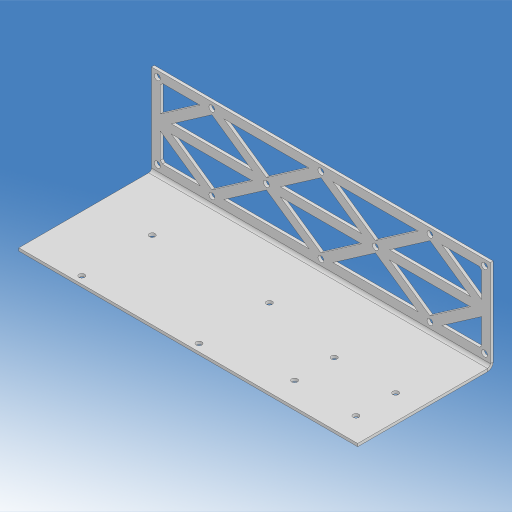
# Autodesk Inventor part: NEMA34_gearbox_sheetMetaMount
Saved by Autodesk Inventor 2024 (Build 280153000, 153)
## iProperties
Created: 2024-03-10
Part Number: NEMA34_gearbox_sheetMetaMount
Material: Generic
Document SubType Name: Sheet Metal
Designer: seene
Density: 1 g/cm^3
Sheet Metal Rule: Default
Appearance: Default
Author: seene
Autodesk Inventor part; units mm, degrees
(part 1 of 2)
ref_plane "YZ Plane" through (0, 0, 0) normal (1, 0, 0) x (0, 1, 0)
ref_plane "XZ Plane" through (0, 0, 0) normal (0, 1, 0) x (-1, 0, 0)
sketch "Sketch1" plane through (0, 0, 0) normal (0, 1, 0) x (-1, 0, 0)
  line L0 (0, 0) -> (144.145, 0) construction
  line L1 (144.145, 0) -> (144.145, -660.4) construction
  line L2 (144.145, -660.4) -> (0, -660.4) construction
  line L3 (0, -660.4) -> (0, 0) construction
  line L4 (144.145, -76.2) -> (0, -76.2) construction
  line L5 (144.145, -584.2) -> (0, -584.2) construction
  circle A0 centre (119.126, -452.5645) radius 3.175
  circle A1 centre (119.126, -519.1125) radius 3.175
  circle A2 centre (76.2, -519.1125) radius 3.175
  line L6 (55.753, -528.8044) -> (55.753, -436.6387) construction
  line L7 (139.573, -436.6387) -> (139.573, -528.8044) construction
  line L8 (55.753, -436.6387) -> (139.573, -436.6387) construction
  circle A3 centre (76.2, -452.5645) radius 3.175
  line L9 (139.573, -528.8044) -> (55.753, -528.8044) construction
  line L10 (92.9069, -436.6387) -> (102.4192, -436.6387) construction
  line L11 (102.4192, -412.6865) -> (92.9069, -412.6865) construction
  line L12 (92.9069, -412.6865) -> (92.9069, -436.6387) construction
  line L13 (97.663, -412.6865) -> (97.663, -436.6387) construction
  line L14 (102.4192, -436.6387) -> (102.4192, -412.6865) construction
  line L15 (89.7255, -412.623) -> (105.6005, -412.623) construction
  line L16 (140.97, -384.048) -> (54.356, -384.048) construction
  line L17 (105.6005, -384.048) -> (89.7255, -384.048) construction
  line L18 (89.7255, -384.048) -> (89.7255, -412.623) construction
  line L19 (97.663, -384.048) -> (97.663, -412.623) construction
  line L20 (105.6005, -412.623) -> (105.6005, -384.048) construction
  line L21 (140.97, -229.616) -> (140.97, -384.048) construction
  line L22 (54.356, -384.048) -> (54.356, -229.616) construction
  circle A4 centre (136.2075, -366.141) radius 3.175
  circle A5 centre (136.2075, -239.141) radius 3.175
  circle A6 centre (60.0075, -239.141) radius 3.175
  line L23 (54.356, -229.616) -> (140.97, -229.616) construction
  circle A7 centre (60.0075, -366.141) radius 3.175
  line L24 (144.145, -178.816) -> (0, -178.816)
  line L25 (0, -178.816) -> (0, -545.9494)
  line L26 (0, -545.9494) -> (144.145, -545.9494)
  line L27 (144.145, -545.9494) -> (144.145, -178.816)
  line L28 (139.573, -479.4885) -> (168.0972, -479.4885) construction
  line L29 (168.0972, -479.4885) -> (168.0972, -492.1885) construction
  line L30 (168.0972, -492.1885) -> (139.573, -492.1885) construction
  line L31 (139.573, -492.1885) -> (139.573, -479.4885) construction
  line L32 (168.0972, -485.8385) -> (139.573, -485.8385) construction
  line L33 (161.3624, -485.8385) -> (168.576, -485.8385) construction
  line L34 (136.4065, -431.8) -> (172.5514, -431.8) construction
  point P0 (89.7255, -398.3355)
  point P1 (72.0725, 0)
  point P2 (72.0725, -660.4)
  point P3 (72.0725, -178.816)
  point P4 (154.479, -431.8)
  dimension "d4" = 76.2
  dimension "d5" = 76.2
  dimension "d6" = 6.35
  dimension "d7" = 66.548
  dimension "d8" = 42.926
  dimension "d9" = 83.82
  dimension "d10" = 92.1657
  dimension "d11" = 20.447
  dimension "d12" = 15.9258
  dimension "d14" = 9.5123
  dimension "d16" = 23.9522
  dimension "d18" = 41.91
  dimension "d19" = 154.432
  dimension "d20" = 86.614
  dimension "d21" = 28.575
  dimension "d23" = 127
  dimension "d24" = 76.2
  dimension "d25" = 4.7625
  dimension "d26" = 9.525
  dimension "d27" = 15.875
  dimension "d28" = 144.145
  dimension "d29" = 660.4
  dimension "d30" = 6.35
  dimension "d116" = 28.5242
  dimension "d117" = 12.7
  dimension "d118" = 49.1998
  dimension "d122" = 50.8
  dimension "d123" = 17.145
  dimension "d126" = 0.0635
  dimension "d130" = 152.4
  dimension "d131" = 54.0385
  dimension "d490" = 3.175
  measures "d4" distance between parallel lines of L0 L4
  measures "d5" distance between parallel lines of L2 L5
  measures "d6" diameter of A0
  measures "d7" distance of A0.centre A1.centre
  measures "d8" distance of A0.centre A3.centre
  measures "d9" distance of L9.start L6.start
  measures "d10" distance of L6.start L8.start
  measures "d11" distance from line of L7 A0.centre
  measures "d12" distance from line of A0.centre L8
  measures "d14" distance of L11.start L11.end
  measures "d16" distance of L10.end L11.start
  measures "d18" distance between parallel lines of L7 L13
  measures "d19" distance of L23.end L21.end
  measures "d20" distance of L23.start L23.end
  measures "d21" distance of L15.end L17.start
  measures "d23" distance of A5.centre A4.centre
  measures "d24" distance of A5.centre A6.centre
  measures "d25" distance from line of L21 A5.centre
  measures "d26" distance from line of A6.centre L23
  measures "d27" distance from line of point (89.726, -398.336) L20
  measures "d28" distance between parallel lines of L3 L1
  measures "d29" distance from line of point (72.073, -660.4) L0
  measures "d30" diameter of A5
  measures "d116" distance of L29.end L30.end
  measures "d117" distance between parallel lines of L30 L28
  measures "d118" distance between parallel lines of L32 L8
  measures "d122" distance between parallel lines of L23 L24
  measures "d123" distance between parallel lines of L26 L9
  measures "d126" distance between parallel lines of L11 L15
  measures "d130" distance between parallel lines of L5 L34
  measures "d131" distance between parallel lines of L32 L34
  measures "d490" distance between parallel lines of L27 L21
extrude "Plate1" add sketch "Sketch1" along normal blind 3.048
ref_plane "Work Plane1" through (6.35, 0, -178.816) normal (1, 0, 0) x (0, 0, -1)
sketch "Sketch2" plane through (6.35, 0, -178.816) normal (1, 0, 0) x (0, 0, -1)
  line L0 (367.1334, 3.048) -> (0, 3.048) projected
  line L1 (0, 0) -> (0, 3.048) projected
  line L2 (0, 0) -> (367.1334, 0) projected
  line L3 (367.1334, 0) -> (367.1334, 3.048) projected
  line L4 (367.1334, 0) -> (0, 0)
  line L5 (0, 0) -> (0, -85.852)
  line L6 (0, -85.852) -> (367.1334, -85.852)
  line L7 (367.1334, -85.852) -> (367.1334, 0)
  point P0 (-178.816, 0)
  dimension "d132" = 88.9
  constraints: 8 end point, 2 parallel, 1 horizontal, 1 perpendicular
  measures "d132" distance between parallel lines of L0 L6
sketch "Sketch3" plane through (0, 0, 0) normal (0, -1, 0) x (1, 0, 0)
  line L0 (0, -178.816) -> (0, -545.9494) projected
  line L1 (0, -545.9494) -> (88.9, -545.9494)
  line L2 (88.9, -545.9494) -> (88.9, -178.816)
  line L3 (88.9, -178.816) -> (0, -178.816)
  line L4 (0, -178.816) -> (0, -545.9494)
  line L5 (0, -545.9494) -> (0, -178.816)
  point P0 (0, 0)
  point P1 (0, -138.2272)
  dimension "d50" = 88.9
  constraints: 10 end point, 3 equal length, 1 horizontal, 1 perpendicular
  measures "d50" distance of L0.start L2.end
sheet face with bend "Face2" sketch "Sketch3" thickness 3.048 toward (0, 1, 0) bend radius 3.048
bend "Bend1"
fold "Fold1" angle 90 bend radius 3.048 thickness 3.048 k factor 0.44 line from (0, 0, -178.816) to (0, 0, -545.9494) line at bend centre moving side (1, 0, 0) folds toward (0, -1, 0)
sketch "Sketch4" plane through (-0.3992, -88.5008, -545.9494) normal (-1, 0, 0) x (0, 0, 1)
  line L0 (367.1334, 85.4528) -> (0, 85.4528) projected
  line L1 (0, 85.4528) -> (0, 0) projected
  line L2 (0, 0) -> (367.1334, 0) projected
  line L3 (367.1334, 0) -> (409.19, 0)
  line L4 (409.19, 0) -> (409.19, 148.9528)
  line L5 (409.19, 148.9528) -> (367.1334, 148.9528)
  line L6 (367.1334, 148.9528) -> (367.1334, 0)
  line L7 (0, 0) -> (-42.7389, 0)
  line L8 (-42.7389, 0) -> (-42.7389, 148.9528)
  line L9 (-42.7389, 148.9528) -> (0, 148.9528)
  line L10 (0, 148.9528) -> (0, 0)
  line L11 (367.1334, 0) -> (-39.2666, 0)
  line L12 (367.1334, 85.4528) -> (367.1334, 0) projected
  point P0 (545.9494, 88.5008)
  constraints: 18 end point, 4 parallel, 3 horizontal, 2 perpendicular
feature "Fold2" [suppressed]
feature "Fold3" [suppressed]
sketch "Sketch5" plane through (-0.3992, -152.0008, -529.9528) normal (-1, 0, 0) x (0, 0, 1)
  line L0 (0, 0) -> (399.5056, 0) projected
  line L1 (399.5056, 0) -> (0, 0)
  line L2 (0, 0) -> (0, -21.8664)
  line L3 (0, -21.8664) -> (399.5056, -21.8664)
  line L4 (399.5056, -21.8664) -> (399.5056, 0)
  point P0 (529.9528, 152.0008)
  constraints: 8 end point, 2 parallel, 1 horizontal, 1 perpendicular
feature "Fold5" [suppressed]
sketch "Sketch6" plane through (5.6968, -91.5488, -178.816) normal (0, -1, 0) x (-1, 0, 0)
  line L0 (0, -367.1334) -> (0, 0)
  line L1 (0, 0) -> (-19.304, 0)
  line L2 (-19.304, 0) -> (-19.304, -367.1334)
  line L3 (-19.304, -367.1334) -> (0, -367.1334)
  constraints: 6 end point, 1 horizontal, 1 perpendicular, 1 vertical
sketch "Sketch7" plane through (5.6968, -88.5008, -548.9974) normal (0, 0, -1) x (1, 0, 0)
  line L0 (0, 85.4528) -> (0, 0)
  line L1 (0, 0) -> (19.304, 0)
  line L2 (19.304, 0) -> (19.304, 85.4528)
  line L3 (19.304, 85.4528) -> (0, 85.4528)
  constraints: 6 end point, 1 horizontal, 1 perpendicular, 1 vertical
sketch "Sketch8" plane through (5.6968, -3.048, -175.768) normal (0, 0, 1) x (-1, 0, 0)
  line L0 (0, -85.4528) -> (0, 0)
  line L1 (0, 0) -> (-19.304, 0)
  line L2 (-19.304, 0) -> (-19.304, -85.4528)
  line L3 (-19.304, -85.4528) -> (0, -85.4528)
  constraints: 6 end point, 1 horizontal, 1 perpendicular, 1 vertical
sketch "Sketch9" plane through (-0.3992, -88.5008, -545.9494) normal (-1, 0, 0) x (0, 0, 1)
  line L0 (0, 0) -> (367.1334, 0)
  line L1 (367.1334, 0) -> (0, 0)
  line L2 (0, 0) -> (0, -9.3726)
  line L3 (0, -9.3726) -> (367.1334, -9.3726)
  line L4 (367.1334, -9.3726) -> (367.1334, 0)
  point P0 (545.9494, 88.5008)
  dimension "d140" = 9.3726
  measures "d140" distance of L1.end L2.end
sheet face with bend "Face5" sketch "Sketch9" thickness 3.048 toward (1, 0, 0) bend radius 3.048
bend "Bend7"
sketch "Sketch13" plane through (-0.3992, -91.5488, -545.9494) normal (0, 1, 0) x (1, 0, 0)
  line L0 (6.096, 6.096) -> (25.4, 6.096) projected
  arc A0 (6.096, 6.096) -> (0, 0) centre (6.096, 0) ccw projected
  line L1 (6.096, 6.096) -> (6.096, 3.048) projected
  line L2 (6.096, 3.048) -> (25.4, 3.048) projected
  line L3 (25.4, 6.096) -> (25.4, 3.048) projected
  line L4 (6.096, 6.096) -> (25.4, 6.096) projected
  line L5 (6.096, 6.096) -> (6.096, 3.048) projected
  arc A1 (6.096, 6.096) -> (0, 0) centre (6.096, 0) ccw projected
  line L6 (3.048, 0) -> (0, 0) projected
  arc A2 (6.096, 3.048) -> (3.048, 0) centre (6.096, 0) ccw projected
  point P0 (0.3992, -545.9494)
  point P1 (0, 0)
extrude "Extrusion1" [suppressed]
sketch "Sketch17" plane through (-0.3992, -97.8734, -545.9494) normal (-1, 0, 0) x (0, 0, 1)
  line L0 (183.3645, 6.35) -> (183.5667, 94.8254) construction
  line L1 (367.1334, 94.8254) -> (0, 94.8254) construction
  line L2 (0, 94.8254) -> (0, 0) construction
  line L3 (0, 0) -> (65.405, 0) construction
  line L4 (65.405, 0) -> (65.405, 6.35) construction
  line L5 (65.405, 6.35) -> (0, 6.35) construction
  line L6 (0, 6.35) -> (0, 0) construction
  circle A0 centre (65.405, 6.35) radius 3.302 construction
  line L7 (0, 0) -> (367.1334, 0) construction
  line L8 (367.1334, 0) -> (0, 0) construction
  line L9 (367.1334, 0) -> (301.7284, 0) construction
  line L10 (301.7284, 0) -> (301.7284, 6.35) construction
  line L11 (301.7284, 6.35) -> (367.1334, 6.35) construction
  line L12 (367.1334, 6.35) -> (367.1334, 0) construction
  circle A1 centre (301.7284, 6.35) radius 3.302 construction
  line L13 (301.7284, 6.35) -> (65.405, 6.35) construction
  line L14 (183.5667, 94.8254) -> (183.5522, 88.4754) construction
  circle A2 centre (183.5522, 88.4754) radius 3.302 construction
  line L15 (301.7284, 6.35) -> (301.7284, 94.8254) construction
  line L16 (65.405, 6.35) -> (65.405, 94.8254) construction
  line L17 (183.5522, 88.4754) -> (367.148, 88.4754) construction
  line L18 (183.5522, 88.4754) -> (0, 88.4754) construction
  circle A3 centre (65.405, 88.4754) radius 3.302 construction
  circle A4 centre (301.7284, 88.4754) radius 3.302 construction
  line L19 (0, 47.4127) -> (367.1334, 47.4127) construction
  line L20 (301.7284, 0) -> (242.5464, 0) construction
  line L21 (242.5464, 0) -> (242.5464, 94.8254) construction
  line L22 (65.405, 0) -> (124.587, 0) construction
  line L23 (124.587, 0) -> (124.587, 94.8254) construction
  circle A5 centre (242.5464, 47.4127) radius 3.302 construction
  circle A6 centre (124.587, 47.4127) radius 3.302 construction
  line L24 (0, 0) -> (6.35, 0) construction
  line L25 (6.35, 0) -> (6.35, 94.8182) construction
  line L26 (6.35, 94.8182) -> (0, 94.8182) construction
  line L27 (0, 94.8182) -> (0, 0) construction
  line L28 (367.1334, 0) -> (360.7834, 0) construction
  line L29 (360.7834, 0) -> (360.7834, 94.8254) construction
  line L30 (360.7834, 94.8254) -> (367.1334, 94.8254) construction
  line L31 (367.1334, 94.8254) -> (367.1334, 0) construction
  line L32 (124.587, 6.35) -> (183.5667, 6.35) construction
  circle A7 centre (183.3645, 6.35) radius 3.302 construction
  line L33 (242.5464, 47.4127) -> (183.3645, 6.35) construction
  line L34 (183.3645, 6.35) -> (124.587, 47.4127) construction
  circle A8 centre (242.5464, 47.4127) radius 6.477 construction
  circle A9 centre (183.3645, 6.35) radius 6.477 construction
  circle A10 centre (124.587, 47.4127) radius 6.477 construction
  circle A11 centre (65.405, 6.35) radius 6.477 construction
  circle A12 centre (65.405, 88.4754) radius 6.477 construction
  circle A13 centre (183.5522, 88.4754) radius 6.477 construction
  circle A14 centre (301.7284, 6.35) radius 6.477 construction
  circle A15 centre (301.7284, 88.4754) radius 6.477 construction
  line L35 (242.5464, 47.4127) -> (301.7284, 88.4754) construction
  line L36 (301.7284, 88.4754) -> (183.5522, 88.4754) construction
  line L37 (183.5522, 88.4754) -> (242.5464, 47.4127) construction
  line L38 (183.5522, 88.4754) -> (124.587, 47.4127) construction
  line L39 (124.587, 47.4127) -> (65.405, 6.35) construction
  line L40 (65.405, 6.35) -> (6.35, 47.4091) construction
  line L41 (65.405, 88.4754) -> (6.35, 47.4091) construction
  line L42 (65.405, 88.4754) -> (124.587, 47.4127) construction
  line L43 (360.7834, 47.4127) -> (301.7284, 6.35) construction
  line L44 (360.7834, 47.4127) -> (301.7284, 88.4754) construction
  line L45 (301.7284, 6.35) -> (301.7284, 6.35) construction
  line L46 (240.9581, 45.1333) -> (303.1759, 8.4442) construction
  line L47 (300.2941, 4.2608) -> (243.8644, 49.299) construction
  line L48 (301.7284, 6.35) -> (301.7284, 6.35) construction
  line L49 (362.2331, 45.3278) -> (359.3334, 49.4981) construction
  line L50 (359.3334, 49.4981) -> (304.9669, 5.7051) construction
  line L51 (300.2788, 8.4349) -> (362.2331, 45.3278) construction
  line L52 (300.2784, 86.39) -> (359.3334, 45.3273) construction
  line L53 (359.3334, 45.3273) -> (362.2335, 49.4981) construction
  line L54 (362.2335, 49.4981) -> (303.1785, 90.5608) construction
  line L55 (303.1785, 90.5608) -> (300.2784, 86.39) construction
  line L56 (300.2784, 86.39) -> (362.2335, 49.4981) construction
  line L57 (359.3334, 45.3273) -> (303.1785, 90.5608) construction
  line L58 (300.2805, 90.5623) -> (241.0985, 49.4996) construction
  line L59 (303.1764, 86.3885) -> (300.2805, 90.5623) construction
  line L60 (300.2805, 90.5623) -> (243.9944, 45.3258) construction
  line L61 (241.0985, 49.4996) -> (303.1764, 86.3885) construction
  line L62 (183.3545, 6.35) -> (183.3452, 6.3635) construction
  line L63 (181.9098, 8.4322) -> (244.0011, 45.3305) construction
  line L64 (241.1052, 49.5042) -> (184.8057, 4.2585) construction
  line L65 (122.9964, 45.4255) -> (125.9057, 49.5899) construction
  line L66 (125.9057, 49.5899) -> (182.0458, 4.1728) construction
  line L67 (184.9551, 8.3372) -> (122.9964, 45.4255) construction
  line L68 (123.1389, 49.4995) -> (63.9572, 8.437) construction
  line L69 (63.9572, 8.437) -> (66.8531, 4.2632) construction
  line L70 (66.8531, 4.2632) -> (126.0348, 45.3257) construction
  line L71 (126.0348, 45.3257) -> (123.1389, 49.4995) construction
  line L72 (123.1389, 49.4995) -> (66.8531, 4.2632) construction
  line L73 (63.9572, 8.437) -> (126.0348, 45.3257) construction
  line L74 (4.9, 45.3236) -> (63.955, 4.2645) construction
  line L75 (63.955, 4.2645) -> (66.855, 8.4355) construction
  line L76 (66.855, 8.4355) -> (7.8, 49.4946) construction
  line L77 (7.8, 49.4946) -> (4.9, 45.3236) construction
  line L78 (4.9, 45.3236) -> (66.855, 8.4355) construction
  line L79 (63.955, 4.2645) -> (7.8, 49.4946) construction
  line L80 (182.1109, 86.3839) -> (185.013, 90.5533) construction
  line L81 (185.013, 90.5533) -> (241.0856, 45.3348) construction
  line L82 (243.9877, 49.5042) -> (182.1109, 86.3839) construction
  line L83 (182.1493, 90.5183) -> (123.094, 49.5435) construction
  line L84 (123.094, 49.5435) -> (125.9899, 45.3698) construction
  line L85 (125.9899, 45.3698) -> (185.0452, 86.3446) construction
  line L86 (185.0452, 86.3446) -> (182.1493, 90.5183) construction
  line L87 (182.1493, 90.5183) -> (125.9899, 45.3698) construction
  line L88 (123.094, 49.5435) -> (185.0452, 86.3446) construction
  line L89 (66.853, 90.5623) -> (126.035, 49.4996) construction
  line L90 (126.035, 49.4996) -> (123.139, 45.3258) construction
  line L91 (123.139, 45.3258) -> (63.957, 86.3885) construction
  line L92 (63.957, 86.3885) -> (66.853, 90.5623) construction
  line L93 (66.853, 90.5623) -> (123.139, 45.3258) construction
  line L94 (126.035, 49.4996) -> (63.957, 86.3885) construction
  line L95 (63.9785, 90.5313) -> (4.8806, 49.527) construction
  line L96 (4.8806, 49.527) -> (7.7765, 45.3532) construction
  line L97 (7.7765, 45.3532) -> (66.8744, 86.3575) construction
  line L98 (66.8744, 86.3575) -> (63.9785, 90.5313) construction
  line L99 (63.9785, 90.5313) -> (7.7765, 45.3532) construction
  line L100 (4.8806, 49.527) -> (66.8744, 86.3575) construction
  line L101 (242.5464, 47.4127) -> (124.587, 47.4127) construction
  line L102 (124.587, 47.4127) -> (6.35, 47.4091) construction
  line L103 (242.5464, 47.4127) -> (360.7834, 47.4127) construction
  line L104 (362.1933, 49.9581) -> (4.94, 49.9473) construction
  line L105 (4.94, 49.9473) -> (4.9402, 44.8673) construction
  line L106 (4.9402, 44.8673) -> (362.1934, 44.8781) construction
  line L107 (362.1934, 44.8781) -> (362.1933, 49.9581) construction
  line L108 (362.1933, 49.9581) -> (4.9402, 44.8673) construction
  line L109 (4.94, 49.9473) -> (362.1934, 44.8781) construction
  line L110 (242.5464, 47.4127) -> (298.8956, 8.0465) construction
  line L111 (301.7284, 6.35) -> (301.7284, 6.35) construction
  line L112 (359.3334, 49.4981) -> (305.1702, 11.8369) construction
  line L113 (302.0107, 9.6399) -> (301.6149, 9.3648) construction
  line L114 (297.2728, 6.35) -> (297.276, 6.3478) construction
  line L115 (301.8382, 9.3635) -> (301.4429, 9.6396) construction
  line L116 (303.8025, 4.7757) -> (303.8924, 4.8382) construction
  line L117 (308.0702, 7.6667) -> (362.2331, 45.3278) construction
  line L118 (246.1685, 42.0431) -> (295.3852, 7.6596) construction
  line L119 (244.0011, 45.3305) -> (243.9978, 45.3282) construction
  line L120 (243.9941, 45.3263) -> (243.9944, 45.3258) construction
  line L121 (244.0008, 45.331) -> (244.0011, 45.3305) construction
  line L122 (241.0985, 49.4996) -> (241.0988, 49.4991) construction
  line L123 (242.5464, 47.4127) -> (242.5465, 47.4126) construction
  line L124 (241.1052, 49.5042) -> (241.1055, 49.5038) construction
  line L125 (242.5464, 47.4127) -> (242.5465, 47.4126) construction
  line L126 (242.5467, 47.4129) -> (242.5464, 47.4125) construction
  line L127 (242.5464, 47.4336) -> (242.5184, 47.3932) construction
  line L128 (241.2113, 45.5153) -> (241.207, 45.5092) construction
  line L129 (243.8671, 49.2972) -> (243.8644, 49.299) construction
  line L130 (185.013, 90.5533) -> (239.1073, 52.9012) construction
  line L131 (242.5464, 50.5074) -> (242.5487, 50.5058) construction
  line L132 (241.2205, 45.5088) -> (241.2163, 45.5028) construction
  line L133 (241.0945, 45.3286) -> (241.0535, 45.2698) construction
  line L134 (297.8823, 11.5614) -> (248.8275, 45.8317) construction
  line L135 (246.5787, 47.4028) -> (246.5645, 47.4127) construction
  line L136 (239.0991, 41.9293) -> (189.7077, 7.6596) construction
  line L137 (183.3694, 9.445) -> (183.3715, 9.4464) construction
  line L138 (186.8118, 11.8334) -> (241.1052, 49.5042) construction
  line L139 (125.9057, 49.5899) -> (179.9348, 11.8444) construction
  line L140 (183.3694, 9.445) -> (183.3715, 9.4435) construction
  line L141 (177.0255, 7.68) -> (122.9964, 45.4255) construction
  line L142 (236.2052, 48.7318) -> (182.1109, 86.3839) construction
  line L143 (248.8897, 48.7223) -> (303.1764, 86.3885) construction
  line L144 (246.9973, 47.4094) -> (247.0021, 47.4127) construction
  line L145 (243.9978, 45.3282) -> (244.0011, 45.3305) construction
  line L146 (245.7279, 46.5286) -> (245.7308, 46.5306) construction
  line L147 (295.2514, 6.35) -> (189.8415, 6.35) construction
  arc A16 (189.8415, 6.35) -> (189.7077, 7.6596) centre (183.3645, 6.35) ccw construction
  arc A17 (295.3852, 7.6596) -> (295.2514, 6.35) centre (301.1322, 6.4109) ccw construction
  arc A18 (239.0991, 41.9293) -> (246.1685, 42.0431) centre (242.5464, 47.4127) ccw construction
  line L148 (295.2514, 6.35) -> (189.8415, 6.35)
  arc A19 (295.3852, 7.6596) -> (295.2514, 6.35) centre (301.1322, 6.4109) ccw
  line L149 (295.3852, 7.6596) -> (246.1685, 42.0431)
  arc A20 (239.0991, 41.9293) -> (246.1685, 42.0431) centre (242.5464, 47.4127) ccw
  line L150 (189.7077, 7.6596) -> (239.0991, 41.9293)
  arc A21 (189.8415, 6.35) -> (189.7077, 7.6596) centre (183.3645, 6.35) ccw
  line L151 (360.7834, 0) -> (360.7834, 94.8254)
  line L152 (360.7834, 6.35) -> (413.3614, 6.35) construction
  arc A22 (308.2054, 6.35) -> (308.0702, 7.6667) centre (301.7284, 6.35) ccw
  line L153 (360.7834, 6.35) -> (360.7834, 44.3198)
  line L154 (308.0702, 7.6667) -> (360.7834, 44.3198)
  line L155 (360.7834, 6.35) -> (308.2054, 6.35)
  arc A23 (308.0703, 87.1594) -> (308.2054, 88.4754) centre (301.7284, 88.4754) ccw
  arc A24 (58.928, 88.4754) -> (59.0702, 87.1257) centre (65.405, 88.4754) ccw
  line L156 (59.0702, 87.1257) -> (6.35, 50.5465)
  line L157 (6.35, 88.4754) -> (6.35, 50.5465)
  line L158 (6.35, 88.4754) -> (58.928, 88.4754)
  arc A25 (305.1702, 11.8369) -> (297.8823, 11.5614) centre (301.7284, 6.35) ccw
  line L159 (352.6887, 44.8778) -> (305.1702, 11.8369)
  line L160 (297.8823, 11.5614) -> (250.1974, 44.8747)
  line L161 (250.1974, 44.8747) -> (352.6887, 44.8778)
  line L162 (234.4322, 44.8742) -> (132.6601, 44.8711)
  line L163 (116.4676, 44.8707) -> (14.6824, 44.8676)
  line L164 (116.4676, 44.8707) -> (68.8523, 11.8334)
  line L165 (61.963, 11.8367) -> (14.6824, 44.8676)
  arc A26 (68.8523, 11.8334) -> (61.963, 11.8367) centre (65.405, 6.35) ccw
  arc A27 (186.8118, 11.8334) -> (179.9348, 11.8444) centre (183.3645, 6.35) ccw
  arc A28 (180.1621, 82.9565) -> (186.9913, 82.9869) centre (183.5522, 88.4754) ccw
  line L166 (186.8118, 11.8334) -> (234.4322, 44.8742)
  line L167 (179.9348, 11.8444) -> (132.6601, 44.8711)
  arc A29 (59.0631, 7.6658) -> (58.928, 6.35) centre (65.405, 6.35) ccw
  line L168 (58.928, 6.35) -> (6.35, 6.35)
  line L169 (6.35, 44.3155) -> (6.35, 6.35)
  line L170 (59.0631, 7.6658) -> (6.35, 44.3155)
  line L171 (176.8875, 6.35) -> (71.882, 6.35)
  line L172 (128.0167, 41.9182) -> (177.0255, 7.68)
  arc A30 (177.0255, 7.68) -> (176.8875, 6.35) centre (183.3645, 6.35) ccw
  arc A31 (71.882, 6.35) -> (71.7482, 7.6596) centre (65.405, 6.35) ccw
  line L173 (121.1397, 41.9293) -> (71.7482, 7.6596)
  arc A32 (121.1397, 41.9293) -> (128.0167, 41.9182) centre (124.587, 47.4127) ccw
  line L174 (308.2054, 88.4754) -> (360.7834, 88.4754)
  line L175 (308.0703, 87.1594) -> (360.7834, 50.5064)
  line L176 (253.8661, 52.1752) -> (298.2811, 82.992)
  line L177 (250.6659, 49.9547) -> (352.6749, 49.9578)
  line L178 (245.9938, 52.8961) -> (295.3852, 87.1658)
  line L179 (239.1073, 52.9012) -> (189.8935, 87.1563)
  arc A33 (245.9938, 52.8961) -> (239.1073, 52.9012) centre (242.5464, 47.4127) ccw
  arc A34 (127.9771, 52.9316) -> (121.1397, 52.8961) centre (124.587, 47.4127) ccw
  arc A35 (61.9925, 82.9703) -> (68.8523, 82.992) centre (65.405, 88.4754) ccw
  line L180 (186.9913, 82.9869) -> (234.4489, 49.9542)
  line L181 (234.4489, 49.9542) -> (132.5928, 49.9511)
  line L182 (132.5928, 49.9511) -> (180.1621, 82.9565)
  line L183 (177.2229, 87.1002) -> (127.9771, 52.9316)
  line L184 (71.882, 88.4754) -> (177.0752, 88.4754)
  line L185 (61.9925, 82.9703) -> (14.3981, 49.9476)
  line L186 (14.3981, 49.9476) -> (116.4735, 49.9507)
  line L187 (68.8523, 82.992) -> (116.4735, 49.9507)
  arc A36 (298.2811, 82.992) -> (305.1702, 82.9886) centre (301.7284, 88.4754) ccw
  line L188 (190.0292, 88.4754) -> (295.2514, 88.4754)
  arc A37 (295.2514, 88.4754) -> (295.3852, 87.1658) centre (301.7284, 88.4754) ccw
  arc A38 (189.8935, 87.1563) -> (190.0292, 88.4754) centre (183.5522, 88.4754) ccw
  line L189 (71.7482, 87.1658) -> (121.1397, 52.8961)
  arc A39 (177.0752, 88.4754) -> (177.2229, 87.1002) centre (183.5522, 88.4754) ccw
  arc A40 (71.7482, 87.1658) -> (71.882, 88.4754) centre (65.405, 88.4754) ccw
  line L190 (257.2591, 42.6524) -> (297.9832, 14.202)
  arc A41 (304.9868, 14.4163) -> (297.9832, 14.202) centre (301.7284, 6.35) ccw
  line L191 (304.9868, 14.4163) -> (345.599, 42.6551)
  line L192 (345.599, 42.6551) -> (257.2591, 42.6524)
  line L193 (358.5609, 40.0675) -> (358.5609, 8.5725)
  line L194 (358.5609, 8.5725) -> (313.2659, 8.5725)
  line L195 (313.2659, 8.5725) -> (358.5609, 40.0675)
  line L196 (290.1978, 8.5725) -> (246.0191, 39.4363)
  arc A42 (239.28, 39.3497) -> (246.0191, 39.4363) centre (242.5464, 47.4127) ccw
  line L197 (239.28, 39.3497) -> (194.9221, 8.5725)
  line L198 (194.9221, 8.5725) -> (290.1978, 8.5725)
  line L199 (139.6951, 52.1739) -> (227.3658, 52.1765)
  line L200 (227.3658, 52.1765) -> (186.8066, 80.4076)
  arc A43 (180.3545, 80.3849) -> (186.8066, 80.4076) centre (183.5522, 88.4754) ccw
  line L201 (180.3545, 80.3849) -> (139.6951, 52.1739)
  line L202 (227.33, 42.6515) -> (139.7219, 42.6489)
  line L203 (139.7219, 42.6489) -> (180.124, 14.4234)
  arc A44 (186.6309, 14.413) -> (180.124, 14.4234) centre (183.3645, 6.35) ccw
  line L204 (186.6309, 14.413) -> (227.33, 42.6515)
  line L205 (362.0522, 52.3311) -> (313.2671, 86.2529)
  line L206 (313.2671, 86.2529) -> (360.7834, 86.2529)
  line L207 (360.7834, 69.292) -> (358.5609, 69.292)
  line L208 (358.5609, 69.292) -> (358.5609, 54.7587)
  line L209 (358.5609, 69.292) -> (358.5609, 86.2529)
  line L210 (365.327, 50.0541) -> (359.8893, 42.2338)
  line L211 (290.1709, 86.2529) -> (245.8129, 55.4757)
  arc A45 (245.8129, 55.4757) -> (239.292, 55.4805) centre (242.5464, 47.4127) ccw
  line L212 (239.292, 55.4805) -> (195.0817, 86.2529)
  line L213 (195.0817, 86.2529) -> (290.1709, 86.2529)
  line L214 (245.2614, 43.4998) -> (239.8315, 51.3256)
  line L215 (239.8315, 51.3256) -> (304.4434, 84.5625) construction
  line L216 (299.0135, 92.3883) -> (245.2614, 43.4998) construction
  line L217 (242.5464, 42.6502) -> (360.7834, 42.6502)
  line L218 (360.7834, 42.6502) -> (360.7834, 52.1752)
  line L219 (242.5464, 52.1752) -> (242.5464, 42.6502)
  line L220 (242.5464, 42.6502) -> (360.7834, 52.1752) construction
  line L221 (360.7834, 42.6502) -> (242.5464, 52.1752) construction
  arc A46 (127.7847, 55.5032) -> (121.3206, 55.4757) centre (124.587, 47.4127) ccw
  line L222 (127.7847, 55.5032) -> (172.103, 86.2529)
  line L223 (172.103, 86.2529) -> (76.9626, 86.2529)
  line L224 (76.9626, 86.2529) -> (121.3206, 55.4757)
  line L225 (76.9626, 8.5725) -> (171.8673, 8.5725)
  line L226 (171.8673, 8.5725) -> (127.8275, 39.3393)
  arc A47 (121.3205, 39.3497) -> (127.8275, 39.3393) centre (124.587, 47.4127) ccw
  line L227 (121.3205, 39.3497) -> (76.9626, 8.5725)
  line L228 (53.9135, 86.2529) -> (8.5725, 54.7936)
  line L229 (8.5725, 54.7936) -> (8.5725, 86.2529)
  line L230 (8.5725, 86.2529) -> (53.9135, 86.2529)
  line L231 (8.5725, 40.0634) -> (8.5725, 8.5725)
  line L232 (8.5725, 8.5725) -> (53.8656, 8.5725)
  line L233 (53.8656, 8.5725) -> (8.5725, 40.0634)
  line L234 (109.3719, 52.1729) -> (21.5004, 52.1703)
  line L235 (21.5004, 52.1703) -> (62.1804, 80.3956)
  arc A48 (62.1804, 80.3956) -> (68.6714, 80.4124) centre (65.405, 88.4754) ccw
  line L236 (68.6714, 80.4124) -> (109.3719, 52.1729)
  line L237 (21.7441, 42.6453) -> (109.3653, 42.6479)
  line L238 (109.3653, 42.6479) -> (68.6715, 14.413)
  arc A49 (68.6715, 14.413) -> (62.1496, 14.4175) centre (65.405, 6.35) ccw
  line L239 (62.1496, 14.4175) -> (21.7441, 42.6453)
  line L240 (358.3834, 52.1752) -> (357.7377, 52.1752)
  line L241 (349.485, 52.1752) -> (253.8661, 52.1752)
  line L242 (349.485, 52.1752) -> (305.1702, 82.9886)
  line L243 (260.968, 54.3977) -> (298.462, 80.4124)
  arc A50 (298.462, 80.4124) -> (304.9868, 80.4091) centre (301.7284, 88.4754) ccw
  line L244 (304.9868, 80.4091) -> (342.3956, 54.3977)
  line L245 (342.3956, 54.3977) -> (260.968, 54.3977)
  point P0 (545.9494, 97.8734)
  point P1 (272.0713, 26.7863)
  point P2 (331.2559, 26.8813)
  point P3 (331.2559, 67.9441)
  point P4 (272.1374, 67.9441)
  point P5 (212.9555, 26.8813)
  point P6 (153.9757, 26.8813)
  point P7 (94.996, 26.8813)
  point P8 (35.8775, 26.8796)
  point P9 (213.0493, 67.9441)
  point P10 (154.0696, 67.9441)
  point P11 (94.996, 67.9441)
  point P12 (35.8775, 67.9423)
  point P13 (183.5667, 47.4127)
  point P14 (272.1374, 67.9441)
  point P15 (301.6649, 47.4127)
  dimension "d298" = 6.604
  dimension "d304" = 12.954
  dimension "d305" = 12.954
  dimension "d310" = 12.954
  dimension "d285" = 65.405
  dimension "d286" = 6.35
  dimension "d287" = 6.604
  dimension "d288" = 65.405
  dimension "d289" = 6.35
  dimension "d290" = 6.604
  dimension "d292" = 6.35
  dimension "d293" = 6.604
  dimension "d294" = 6.604
  dimension "d295" = 6.604
  dimension "d296" = 59.182
  dimension "d297" = 59.182
  dimension "d299" = 6.604
  dimension "d300" = 6.35
  dimension "d301" = 94.8182
  dimension "d302" = 6.35
  dimension "d303" = 6.604
  dimension "d306" = 12.954
  dimension "d307" = 12.954
  dimension "d308" = 12.954
  dimension "d309" = 12.954
  dimension "d311" = 12.954
  dimension "d312" = 5.08
  dimension "d313" = 5.08
  dimension "d314" = 5.08
  dimension "d315" = 5.08
  dimension "d316" = 5.08
  dimension "d317" = 5.08
  dimension "d318" = 5.08
  dimension "d319" = 5.08
  dimension "d320" = 5.08
  dimension "d321" = 5.08
  dimension "d322" = 5.08
  dimension "d323" = 5.08
  dimension "d324" = 5.08
  dimension "d335" = 5.0793
  dimension "d336" = 2.2225
  dimension "d337" = 2.2225
  dimension "d338" = 2.2225
  dimension "d339" = 2.2225
  dimension "d340" = 2.2225
  dimension "d341" = 2.2225
  dimension "d342" = 2.2225
  dimension "d344" = 2.2225
  dimension "d345" = 9.525
  dimension "d346" = 9.525
  dimension "d347" = 2.2225
  dimension "d348" = 2.2225
  dimension "d349" = 2.2225
  dimension "d350" = 2.2225
  dimension "d351" = 2.2225
  dimension "d352" = 2.2225
  dimension "d353" = 2.2225
  constraints: 484 end point, 125 point on line, 101 point on circle, 82 parallel, 50 midpoint, 47 centre point, 38 perpendicular, 19 collinear, 12 concentric, 9 coincident, 9 horizontal, 1 vertical, 86 other
  measures "d285" distance of L5.end L4.end
  measures "d286" distance of L4.end L3.end
  measures "d287" diameter of A0
  measures "d288" distance of L10.end L11.end
  measures "d289" distance of L10.end L9.end
  measures "d290" diameter of A1
  measures "d292" distance of L0.end L14.end
  measures "d293" diameter of A2
  measures "d294" diameter of A3
  measures "d295" diameter of A4
  measures "d296" distance of L9.end L20.end
  measures "d297" distance of L3.end L22.end
  measures "d299" diameter of A6
  measures "d300" distance of L26.end L25.end
  measures "d301" distance of L25.end L24.end
  measures "d302" distance of L29.end L30.end
  measures "d303" diameter of A7
  measures "d306" diameter of A10
  measures "d307" diameter of A11
  measures "d308" diameter of A12
  measures "d309" diameter of A13
  measures "d311" diameter of A15
  measures "d312" distance of L46.end L47.start
  measures "d313" distance of L116.start L51.start
  measures "d314" distance of L53.end L52.end
  measures "d315" distance of L60.end L58.end
  measures "d316" distance of L63.end L64.start
  measures "d317" distance of L67.start L66.end
  measures "d318" distance of L69.end L68.end
  measures "d319" distance of L75.end L74.end
  measures "d320" distance of L82.start L81.end
  measures "d321" distance of L84.end L83.end
  measures "d322" distance of L89.end L90.end
  measures "d323" distance of L96.end L95.end
  measures "d324" distance of L105.end L104.end
  measures "d335" distance between parallel lines of L159 L154
  measures "d336" distance between parallel lines of L160 L190
  measures "d337" distance between parallel lines of L154 L195
  measures "d338" distance between parallel lines of L118 L196
  measures "d339" distance between parallel lines of L181 L199
  measures "d340" distance between parallel lines of L166 L204
  measures "d341" distance between parallel lines of L175 L205
  measures "d342" distance of L207.start L207.end
  measures "d344" distance between parallel lines of L178 L211
  measures "d345" distance of L216.start L215.end
  measures "d346" distance of L218.end L217.end
  measures "d347" radial gap between concentric circles of A34 A46
  measures "d348" distance between parallel lines of L173 L227
  measures "d349" distance between parallel lines of L158 L230
  measures "d350" distance between parallel lines of L170 L233
  measures "d351" distance between parallel lines of L187 L236
  measures "d352" distance between parallel lines of L165 L239
  measures "d353" distance between parallel lines of L241 L245
cut "Cut2" [suppressed]
hole "Hole5" [suppressed]
sketch "Sketch20" plane through (-0.3992, -88.5008, -545.9494) normal (-1, 0, 0) x (0, 0, 1)
  point P0 (545.9494, 88.5008)